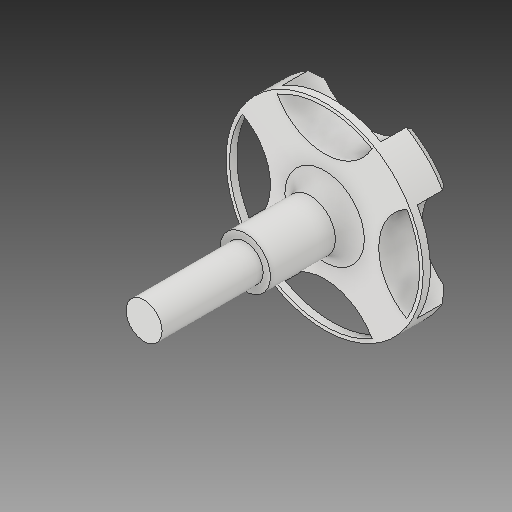
# Autodesk Inventor part: Motor Bot
Saved by Autodesk Inventor 2019.1 (Build 231200000, 200)
## iProperties
Created: 2018-12-11
Part Number: Motor Bot
Material: ABS Plastic
Document SubType Name: Modeling
Designer: Kanenas
Density: 1.06 g/cm^3
Appearance: Smooth - White
Author: Kanenas
Autodesk Inventor part; units mm, degrees
ref_plane "YZ Plane" through (0, 0, 0) normal (1, 0, 0) x (0, 1, 0)
ref_plane "XZ Plane" through (0, 0, 0) normal (0, 1, 0) x (-1, 0, 0)
ref_plane "XY Plane" through (0, 0, 0) normal (0, 0, 1) x (1, 0, 0)
sketch "Sketch1" plane through (0, 0, 0) normal (0, 0, 1) x (1, 0, 0)
  circle A0 centre (0, 0) radius 13.65
  dimension "d0" = 27.3
  constraints: 1 centre point, 1 coincident
  measures "d0" diameter of A0
extrude "Extrusion1" add sketch "Sketch1" along normal blind 5
sketch "Sketch2" plane through (0, 0, 0) normal (0, 0, -1) x (-1, 0, 0)
  circle A0 centre (0, 0) radius 9.5 construction
  circle A1 centre (0, 0) radius 8 construction
  circle A2 centre (5.6569, 5.6569) radius 1.5
  line L0 (0, 0) -> (5.6569, 5.6569)
  line L1 (0, 0) -> (15.4714, 0)
  circle A3 centre (-6.7175, 6.7175) radius 1.5
  line L2 (-6.7175, 6.7175) -> (0, 0)
  dimension "d3" = 19
  dimension "d4" = 16
  dimension "d5" = 3
  dimension "d6" = 45
  dimension "d41" = 3
  dimension "d42" = 90
  constraints: 6 end point, 3 coincident, 2 centre point, 1 horizontal, 6 other
  measures "d5" diameter of A2
  measures "d6" angle of L1 L0
  measures "d41" diameter of A3
  measures "d42" angle of L2 L0
extrude "Extrusion2" cut sketch "Sketch2" against normal blind 16.03
pattern_circular "Circular Pattern1" count 2 over 360 about axis through (0, 0, -10) along (0, 0, 1) of "Extrusion2"
chamfer "Chamfer1" distance 1.5 angle 45 1 edges at (-13.65, 0, 0)
sketch "Sketch3" plane through (0, 0, 0) normal (0, 0, -1) x (-1, 0, 0)
  circle A0 centre (15, 0) radius 7.5
  point P0 (0, 0)
  dimension "d15" = 15
  dimension "d16" = 15
  constraints: 1 centre point
  measures "d15" diameter of A0
  measures "d16" distance of point (0, 0) A0.centre
extrude "Extrusion3" cut sketch "Sketch3" against normal blind 54.97
pattern_circular "Circular Pattern2" count 4 over 360 about axis through (0, 0, -10) along (0, 0, 1) of "Extrusion3"
shell "Shell1" thickness 1 removed faces 3 at (0.0902, 2.5799, 5) at (7.1374, -5.4162, 3.3333) at (-7.1374, 5.4162, 3.3333)
sketch "Sketch4" plane through (0, 0, 5) normal (0, 0, 1) x (1, 0, 0)
  circle A0 centre (0, 0) radius 13.65
  dimension "d23" = 27.3
  constraints: 1 centre point, 1 coincident
  measures "d23" diameter of A0
extrude "Extrusion4" add sketch "Sketch4" along normal blind 1
sketch "Sketch6" plane through (0, 0, 5) normal (0, 0, -1) x (-1, 0, 0)
  arc A0 (-6.5735, -11.3891) -> (6.5735, -11.3891) centre (0, 0) ccw
  arc A1 (6.5735, -11.3891) -> (-6.5735, -11.3891) centre (0, -15) ccw
  dimension "d30" = 26.3
  dimension "d31" = 15
  dimension "d32" = 15
  constraints: 4 point on circle, 2 centre point, 1 coincident
  measures "d30" diameter of A0
  measures "d31" distance of point (0, 0) A1.centre
  measures "d32" diameter of A1
extrude "Extrusion6" cut sketch "Sketch6" against normal blind 12.03
sketch "Sketch5" plane through (0, 0, 6) normal (0, 0, 1) x (1, 0, 0)
  circle A0 centre (0, 0) radius 3.5
  dimension "d26" = 7
  constraints: 1 centre point, 1 coincident
  measures "d26" diameter of A0
extrude "Extrusion5" add sketch "Sketch5" along normal blind 11
fillet "Fillet1" radius 2 1 edges at (-3.5, 0, 6)
pattern_circular "Circular Pattern3" count 4 over 360 about axis through (0, 0, -10) along (0, 0, 1) of "Extrusion6"
sketch "Sketch7" plane through (0, 0, 17) normal (0, 0, 1) x (1, 0, 0)
  circle A0 centre (0, 0) radius 2.5
  dimension "d38" = 5
  constraints: 1 centre point, 1 coincident
  measures "d38" diameter of A0
extrude "Extrusion7" add sketch "Sketch7" along normal blind 14
body "Solid1"
